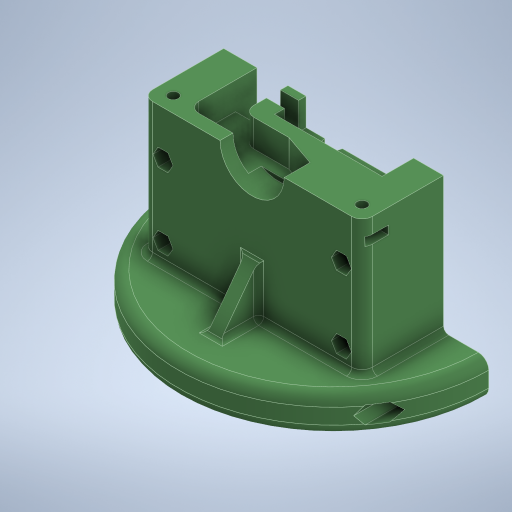
# Autodesk Inventor part: Base_1L
Saved by Autodesk Inventor 2023 (Build 270158000, 158)
## iProperties
Created: 2024-07-30
Part Number: Base_1L
Material: Generic
Document SubType Name: Modeling
Designer: Swoby
Density: 1 g/cm^3
Appearance: Default
Author: Swoby
Autodesk Inventor part; units mm, degrees
ref_plane "YZ Plane" through (0, 0, 0) normal (1, 0, 0) x (0, 1, 0)
ref_plane "XZ Plane" through (0, 0, 0) normal (0, 1, 0) x (-1, 0, 0)
ref_plane "XY Plane" through (0, 0, 0) normal (0, 0, 1) x (1, 0, 0)
sketch "Sketch1" plane through (0, 0, 0) normal (0, 0, 1) x (1, 0, 0)
  arc A0 (-42.5, 0) -> (42.5, 0) centre (0, 0) ccw
  line L0 (-42.5, 0) -> (-42.5, -52.5)
  line L1 (-42.5, -52.5) -> (42.5, -52.5)
  line L2 (42.5, -52.5) -> (42.5, 0)
  line L3 (-42.5, 0) -> (42.5, 0)
  arc A1 (42.5, 0) -> (-42.5, 0) centre (0, 0) ccw construction
  dimension "d0" = 85
  dimension "d1" = 52.5
  constraints: 8 end point, 4 point on circle, 3 perpendicular, 2 centre point, 2 tangent, 1 coincident, 1 vertical
  measures "d0" diameter of A0
  measures "d1" distance from line of L1 point (0, 0)
extrude "Extrusion1" add sketch "Sketch1" along normal blind 31.5
sketch "Sketch2" plane through (-42.5, 0, 0) normal (0, 1, 0) x (1, 0, 0)
  line L0 (31.85, -43.7) -> (73.45, -43.7)
  line L1 (73.45, -3.1) -> (31.85, -3.1)
  line L2 (35.1, -3.1) -> (49.9, -3.1)
  line L3 (49.9, -3.1) -> (49.9, -1.6)
  line L4 (49.9, -1.6) -> (35.1, -1.6)
  line L5 (35.1, -1.6) -> (35.1, -3.1)
  line L6 (37.5, -1.6) -> (47.5, -1.6)
  line L7 (47.5, -1.6) -> (47.5, 0)
  line L8 (47.5, 0) -> (37.5, 0)
  line L9 (37.5, 0) -> (37.5, -1.6)
  line L10 (85, 0) -> (0, 0) projected
  line L11 (31.85, -10.6) -> (24.75, -10.6)
  line L12 (24.75, -10.6) -> (24.75, -14.3)
  line L13 (24.75, -14.3) -> (31.85, -14.3)
  line L14 (73.45, -14.3) -> (80.55, -14.3)
  line L15 (80.55, -14.3) -> (80.55, -10.6)
  line L16 (80.55, -10.6) -> (73.45, -10.6)
  line L17 (31.85, -3.1) -> (31.85, -10.6)
  line L18 (73.45, -43.7) -> (73.45, -14.3)
  line L19 (73.45, -10.6) -> (73.45, -3.1)
  line L20 (31.85, -39.8) -> (25.85, -39.8)
  line L21 (25.85, -39.8) -> (25.85, -34.4)
  line L22 (25.85, -34.4) -> (31.85, -34.4)
  line L23 (31.85, -34.4) -> (31.85, -39.8) construction
  line L24 (31.85, -14.3) -> (31.85, -34.4)
  line L25 (31.85, -39.8) -> (31.85, -43.7)
  point P0 (42.5, 0)
  point P1 (49.9, -2.35)
  point P2 (42.5, -1.6)
  point P3 (42.5, -3.1)
  point P4 (42.5, 0)
  dimension "d4" = 14.8
  dimension "d5" = 1.5
  dimension "d6" = 10
  dimension "d7" = 1.6
  dimension "d9" = 41.6
  dimension "d10" = 40.6
  dimension "d11" = 7.5
  dimension "d12" = 3.7
  dimension "d13" = 7.1
  dimension "d14" = 7.1
  dimension "d15" = 10.65
  dimension "d16" = 3.9
  dimension "d17" = 5.4
  dimension "d18" = 6
  constraints: 50 end point, 15 parallel, 7 perpendicular, 6 horizontal, 6 midpoint, 4 point on line, 3 collinear
  measures "d4" distance from line of point (49.9, -2.35) L5
  measures "d5" distance of L2.end L3.end
  measures "d6" distance between parallel lines of L7 L9
  measures "d7" distance of L6.end L7.end
  measures "d9" distance of L1.start L1.end
  measures "d10" distance of L0.end L1.start
  measures "d11" distance of L1.end L11.start
  measures "d12" distance of L11.end L12.end
  measures "d13" distance of L11.start L11.end
  measures "d14" distance of L15.end L16.end
  measures "d15" distance from line of L17 point (42.5, -3.1)
  measures "d16" distance between parallel lines of L0 L20
  measures "d17" distance of L20.end L21.end
  measures "d18" distance of L21.end L22.end
sketch "Sketch4" plane through (-42.5, -52.5, 0) normal (0, -1, 0) x (1, 0, 0)
  line L0 (0, 31.5) -> (85, 31.5) projected
  arc A0 (-17.5, 31.5) -> (102.5, 31.5) centre (42.5, 31.5) ccw
  line L1 (102.5, 31.5) -> (-17.5, 31.5)
  arc A1 (102.5, 31.5) -> (-17.5, 31.5) centre (42.5, 31.5) ccw construction
  point P0 (42.5, 0)
  dimension "d26" = 120
  constraints: 4 point on circle, 3 midpoint, 2 centre point, 2 end point, 1 horizontal
  measures "d26" diameter of A0
extrude "Extrusion3" add sketch "Sketch4" along normal blind 14
sketch "Sketch5" plane through (0, 0, 31.5) normal (0, 0, 1) x (1, 0, 0)
  line L0 (-34.5, -17.6) -> (34.5, -17.6) construction
  line L1 (34.5, -17.6) -> (34.5, -45.5) construction
  line L2 (34.5, -45.5) -> (-34.5, -45.5) construction
  line L3 (-34.5, -45.5) -> (-34.5, -17.6) construction
  line L4 (-42.5, -52.5) -> (-60, -52.5) projected
  line L5 (-42.5, 0) -> (-42.5, -52.5) projected
  line L6 (42.5, -52.5) -> (42.5, 0) projected
  circle A0 centre (-34.5, -17.6) radius 2
  circle A1 centre (-34.5, -45.5) radius 2
  circle A2 centre (34.5, -45.5) radius 2
  circle A3 centre (34.5, -17.6) radius 2
  line L7 (-60, -52.5) -> (-60, -66.5) projected
  line L8 (60, -66.5) -> (-60, -66.5) projected
  line L9 (60, -52.5) -> (60, -66.5) projected
  line L10 (60, -52.5) -> (42.5, -52.5) projected
  line L11 (42.5, 0) -> (-42.5, 0) projected
  line L12 (42.5, 0) -> (-42.5, 0) projected
  line L13 (-60, -59.5) -> (60, -59.5) construction
  circle A4 centre (-50, -59.5) radius 2
  circle A5 centre (50, -59.5) radius 2
  point P0 (0, 0)
  dimension "d29" = 7
  dimension "d31" = 8
  dimension "d32" = 8
  dimension "d33" = 4
  dimension "d34" = 4
  dimension "d35" = 4
  dimension "d36" = 4
  dimension "d71" = 4
  dimension "d72" = 4
  dimension "d73" = 10
  dimension "d74" = 10
  dimension "d80" = 17.6
  constraints: 10 end point, 6 centre point, 4 coincident, 3 midpoint, 2 parallel, 2 point on line, 1 horizontal, 1 perpendicular
  measures "d29" distance between parallel lines of L4 L2
  measures "d31" distance between parallel lines of L5 L3
  measures "d32" distance between parallel lines of L6 L1
  measures "d33" diameter of A0
  measures "d34" diameter of A1
  measures "d35" diameter of A2
  measures "d36" diameter of A3
  measures "d71" diameter of A4
  measures "d72" diameter of A5
  measures "d73" distance from line of L7 A4.centre
  measures "d74" distance from line of L9 A5.centre
  measures "d80" distance from line of L11 L0.start
extrude "Extrusion4" cut sketch "Sketch5" against normal through all contours A0 | A1 | A2 | A3 | A4 | A5
ref_plane "Work Plane1" through (0, 0, 25.5) normal (0, 0, 1) x (1, 0, 0)
sketch "Sketch6" plane through (0, 0, 25.5) normal (0, 0, 1) x (1, 0, 0)
  circle A0 centre (-34.5, -17.6) radius 2 projected
  circle A1 centre (-34.5, -45.5) radius 2 projected
  circle A2 centre (34.5, -17.6) radius 2 projected
  circle A3 centre (34.5, -45.5) radius 2 projected
  circle A4 centre (-50, -59.5) radius 2 projected
  circle A5 centre (50, -59.5) radius 2 projected
  circle A6 centre (-34.5, -17.6) radius 2 projected
  circle A7 centre (-34.5, -17.6) radius 2 projected
  line L0 (-32.5659, -14.25) -> (-30.6318, -17.6)
  line L1 (-30.6318, -17.6) -> (-32.5659, -20.95)
  line L2 (-32.5659, -20.95) -> (-36.4341, -20.95)
  line L3 (-36.4341, -20.95) -> (-38.3682, -17.6)
  line L4 (-38.3682, -17.6) -> (-36.4341, -14.25)
  line L5 (-36.4341, -14.25) -> (-32.5659, -14.25)
  line L6 (-32.5659, -42.15) -> (-30.6318, -45.5)
  line L7 (-30.6318, -45.5) -> (-32.5659, -48.85)
  line L8 (-32.5659, -48.85) -> (-36.4341, -48.85)
  line L9 (-36.4341, -48.85) -> (-38.3682, -45.5)
  line L10 (-38.3682, -45.5) -> (-36.4341, -42.15)
  line L11 (-36.4341, -42.15) -> (-32.5659, -42.15)
  line L12 (-46.1318, -59.5) -> (-48.0659, -62.85)
  line L13 (-48.0659, -62.85) -> (-51.9341, -62.85)
  line L14 (-51.9341, -62.85) -> (-53.8682, -59.5)
  line L15 (-53.8682, -59.5) -> (-51.9341, -56.15)
  line L16 (-51.9341, -56.15) -> (-48.0659, -56.15)
  line L17 (-48.0659, -56.15) -> (-46.1318, -59.5)
  line L18 (38.3682, -45.5) -> (36.4341, -48.85)
  line L19 (36.4341, -48.85) -> (32.5659, -48.85)
  line L20 (32.5659, -48.85) -> (30.6318, -45.5)
  line L21 (30.6318, -45.5) -> (32.5659, -42.15)
  line L22 (32.5659, -42.15) -> (36.4341, -42.15)
  line L23 (36.4341, -42.15) -> (38.3682, -45.5)
  line L24 (53.8682, -59.5) -> (51.9341, -62.85)
  line L25 (51.9341, -62.85) -> (48.0659, -62.85)
  line L26 (48.0659, -62.85) -> (46.1318, -59.5)
  line L27 (46.1318, -59.5) -> (48.0659, -56.15)
  line L28 (48.0659, -56.15) -> (51.9341, -56.15)
  line L29 (51.9341, -56.15) -> (53.8682, -59.5)
  line L30 (36.4341, -14.25) -> (38.3682, -17.6)
  line L31 (38.3682, -17.6) -> (36.4341, -20.95)
  line L32 (36.4341, -20.95) -> (32.5659, -20.95)
  line L33 (32.5659, -20.95) -> (30.6318, -17.6)
  line L34 (30.6318, -17.6) -> (32.5659, -14.25)
  line L35 (32.5659, -14.25) -> (36.4341, -14.25)
  line L36 (60, -66.5) -> (-60, -66.5) projected
  line L37 (-60, -66.5) -> (60, -66.5) projected
  point P0 (0, 0)
  point P1 (-50, -62.85)
  point P2 (-50, -56.15)
  point P3 (-34.5, -48.85)
  point P4 (-34.5, -42.15)
  point P5 (50, -62.85)
  point P6 (50, -56.15)
  dimension "d85" = 6.7
  dimension "d86" = 6.7
  dimension "d87" = 6.7
  dimension "d88" = 6.7
  dimension "d89" = 6.7
  constraints: 72 end point, 6 coincident, 6 midpoint, 6 parallel, 1 point on line, 80 other
  measures "d85" distance of point (-50, -62.85) point (-50, -56.15)
  measures "d86" distance of point (-34.5, -48.85) point (-34.5, -42.15)
  measures "d87" distance between parallel lines of L2 L5
  measures "d88" distance between parallel lines of L19 L22
  measures "d89" distance of point (50, -62.85) point (50, -56.15)
extrude "Extrusion5" cut sketch "Sketch6" against normal through all contours A0 | A1 | A2 | A3 | A4 | A5 | L0 L1 L2 L3 L4 L5 | L6 L7 L8 L9 L10 L11 | L12 L13 L14 L15 L16 L17 | L18 L19 L20 L21 L22 L23 | L24 L25 L26 L27 L28 L29 | L30 L31 L32 L33 L34 L35
sketch "Sketch7" plane through (-42.5, 0, 31.5) normal (0, 1, 0) x (1, 0, 0)
  line L0 (85, 0) -> (0, 0) projected
  line L1 (85, 31.5) -> (0, 31.5) projected
  line L2 (85, 31.5) -> (0, 31.5) projected
  line L3 (85, 0) -> (0, 0) projected
  circle A0 centre (6, 25.5) radius 2
  circle A1 centre (6, 6) radius 2 construction
  circle A2 centre (79, 25.5) radius 2
  circle A3 centre (79, 6) radius 2 construction
  line L4 (85, 31.5) -> (85, 0) projected
  line L5 (0, 31.5) -> (0, 0) projected
  point P0 (42.5, 31.5)
  dimension "d46" = 4
  dimension "d47" = 4
  dimension "d48" = 4
  dimension "d49" = 4
  dimension "d50" = 6
  dimension "d52" = 6
  dimension "d54" = 6
  dimension "d56" = 6
  dimension "d81" = 6
  dimension "d82" = 6
  constraints: 4 centre point
  measures "d46" diameter of A0
  measures "d47" diameter of A1
  measures "d48" diameter of A2
  measures "d49" diameter of A3
  measures "d50" distance from line of L1 A2.centre
  measures "d52" distance from line of L0 A3.centre
  measures "d54" distance from line of L2 A0.centre
  measures "d56" distance from line of L3 A1.centre
  measures "d81" distance from line of L5 A0.centre
  measures "d82" distance from line of L4 A2.centre
extrude "Extrusion6" cut sketch "Sketch7" against normal blind 10 contours A0 | A2
ref_plane "Work Plane2" through (42.5, -6, 31.5) normal (0, 1, 0) x (1, 0, 0)
sketch "Sketch8" plane through (42.5, -6, 31.5) normal (0, 1, 0) x (1, 0, 0)
  circle A0 centre (-79, 25.5) radius 2 construction
  line L0 (-75.65, 23.5659) -> (-79, 21.6318) construction
  line L1 (-79, 21.6318) -> (-82.35, 23.5659) construction
  line L2 (-82.35, 23.5659) -> (-82.35, 27.4341) construction
  line L3 (-82.35, 27.4341) -> (-79, 29.3682) construction
  line L4 (-79, 29.3682) -> (-75.65, 27.4341) construction
  line L5 (-75.65, 27.4341) -> (-75.65, 23.5659) construction
  line L6 (-75.35, 27.6073) -> (-79, 29.7147)
  line L7 (-79, 29.7147) -> (-82.65, 27.6073)
  line L8 (-82.65, 27.6073) -> (-82.65, 23.3927)
  line L9 (-82.65, 23.3927) -> (-79, 21.2853)
  line L10 (-79, 21.2853) -> (-75.35, 23.3927)
  line L11 (-75.35, 23.3927) -> (-75.35, 27.6073)
  line L12 (17.5, 0) -> (-102.5, 0) projected
  arc A1 (17.5, 0) -> (-102.5, 0) centre (-42.5, 0) ccw projected
  line L13 (0, 31.5) -> (-85, 31.5) projected
  line L14 (-85, 31.5) -> (0, 31.5) projected
  line L15 (-85, 31.5) -> (-85, 0) projected
  line L16 (-85, 31.5) -> (-85, 0) projected
  line L17 (0, 31.5) -> (0, 0) projected
  line L18 (0, 31.5) -> (0, 0) projected
  line L19 (-6, 0) -> (-10, 0) projected
  line L20 (-75, 0) -> (-79, 0) projected
  line L21 (-6, 0) -> (-10, 0) projected
  line L22 (-75, 0) -> (-79, 0) projected
  line L23 (0, 0) -> (-85, 0) projected
  line L24 (-85, 0) -> (-102.5, 0) projected
  line L25 (17.5, 0) -> (-102.5, 0) projected
  line L26 (17.5, 0) -> (0, 0) projected
  line L27 (-6, 21.2853) -> (0, 21.2853)
  line L28 (-6, 29.7147) -> (0, 29.7147)
  line L29 (0, 21.2853) -> (0, 29.7147)
  line L30 (-79, 29.7147) -> (-85, 29.7147)
  line L31 (-85, 29.7147) -> (-85, 21.2853)
  line L32 (-79, 21.2853) -> (-85, 21.2853)
  line L33 (-9.35, 27.4341) -> (-6, 29.3682) construction
  line L34 (-6, 29.3682) -> (-2.65, 27.4341) construction
  line L35 (-2.65, 27.4341) -> (-2.65, 23.5659) construction
  line L36 (-2.65, 23.5659) -> (-6, 21.6318) construction
  line L37 (-6, 21.6318) -> (-9.35, 23.5659) construction
  line L38 (-9.35, 23.5659) -> (-9.35, 27.4341) construction
  line L39 (-9.65, 27.6073) -> (-6, 29.7147)
  line L40 (-6, 29.7147) -> (-2.35, 27.6073)
  line L41 (-2.35, 27.6073) -> (-2.35, 23.3927)
  line L42 (-2.35, 23.3927) -> (-6, 21.2853)
  line L43 (-6, 21.2853) -> (-9.65, 23.3927)
  line L44 (-9.65, 23.3927) -> (-9.65, 27.6073)
  point P0 (-42.5, 31.5)
  point P1 (-6, 25.5)
  point P2 (-11.75, 31.5)
  point P3 (-4.25, 31.5)
  point P4 (-80.75, 31.5)
  point P5 (-73.25, 31.5)
  point P6 (-11.75, 31.5)
  point P7 (-4.25, 31.5)
  point P8 (-80.75, 31.5)
  point P9 (-73.25, 31.5)
  point P10 (-6, 25.5)
  point P11 (-2.65, 25.5)
  dimension "d65" = 0.3
  dimension "d70" = 6.7
  dimension "d83" = 6.7
  dimension "d84" = 0.3
  constraints: 60 end point, 6 point on line, 3 perpendicular, 2 coincident, 2 parallel, 1 midpoint, 36 other
  measures "d65" distance between parallel lines of L4 L6
  measures "d70" distance between parallel lines of L2 L5
  measures "d83" distance from line of point (-2.65, 25.5) L38
  measures "d84" distance between parallel lines of L38 L44
extrude "Extrusion7" cut sketch "Sketch8" against normal blind 3.3 contours L11 L10 L9 L8 L7 L6 | L7 L8 L9 L32 L15 L30 | L17 L27 L42 L41 L40 L28 | L40 L41 L42 L43 L44 L39
fillet "Fillet1" radius 4 4 edges at (0, -52.5, -28.5) (42.5, -26.25, 0) (-42.5, -26.25, 0) (0, -66.5, -28.5)
mirror "Mirror1" about plane through (0, -26.25, 31.5) normal (0, 0, 1) remove original yes
extrude "Extrusion8" cut sketch "Sketch2" against normal blind 10.6 contours L25 L20 L21 L22 L24 L13 L12 L11 L17 L1 L19 L16 L15 L14 L18 L0
sketch "Sketch9" plane through (-38.5, 0, 63) normal (0, 1, 0) x (1, 0, 0)
  line L0 (27.85, 31.5) -> (69.45, 31.5) projected
  line L1 (27.85, 28.6) -> (27.85, 31.5) projected
  line L2 (21.85, 28.6) -> (27.85, 28.6) projected
  line L3 (21.85, 23.2) -> (21.85, 28.6) projected
  line L4 (27.85, 23.2) -> (21.85, 23.2) projected
  line L5 (27.85, 19.3) -> (27.85, 23.2) projected
  line L6 (69.45, 19.3) -> (27.85, 19.3) projected
  line L7 (69.45, 31.5) -> (69.45, 19.3) projected
  line L8 (21.85, 23.2) -> (8.85, 23.2)
  line L9 (8.85, 23.2) -> (8.85, 31.5)
  line L10 (8.85, 31.5) -> (20.85, 31.5)
  line L11 (20.85, 31.5) -> (20.85, 28.6)
  line L12 (20.85, 28.6) -> (21.85, 28.6)
  point P0 (38.5, 63)
  dimension "d90" = 12
  dimension "d91" = 1
  constraints: 10 end point, 4 perpendicular, 1 horizontal, 1 point on line
  measures "d90" distance of L9.end L10.end
  measures "d91" distance of L11.end L2.start
extrude "Extrusion9" cut sketch "Sketch9" against normal through all contours L3 L8 L9 L10 L11 L12
sketch "Sketch10" plane through (-38.5, 0, 63) normal (0, 1, 0) x (1, 0, 0)
  line L0 (77, 0) -> (0, 0) projected
  line L1 (38.5, 0) -> (38.5, 15.8762)
  line L2 (38.5, 0) -> (50.9, 0)
  line L3 (50.9, 0) -> (50.9, 10)
  line L4 (50.9, 10) -> (38.5, 10)
  line L5 (38.5, 10) -> (38.5, 0)
  point P0 (38.5, 63)
  point P1 (38.5, 10)
  dimension "d94" = 24.8
  dimension "d95" = 10
  constraints: 10 end point, 2 parallel, 1 horizontal, 1 midpoint, 1 perpendicular, 1 vertical
  measures "d94" diameter of L3 L1
  measures "d95" distance of L2.end L3.end
revolve "Revolution2" cut sketch "Sketch10" angle 360 about axis through (0, 0, 63) along (0, 0, -1)
sketch "Sketch11" plane through (42.5, 0, 59) normal (0, 1, 0) x (1, 0, 0)
  line L0 (-30.1, 6) -> (-30.1, -4) projected
  line L1 (-4, -4) -> (-30.1, -4) projected
  arc A0 (-4, -4) -> (0, 0) centre (-4, 0) ccw projected
  line L2 (0, 0) -> (0, 27.5) projected
  line L3 (0, 27.5) -> (-11.55, 27.5) projected
  line L4 (-11.55, 27.5) -> (-11.55, 15.3) projected
  line L5 (-11.55, 15.3) -> (-53.15, 15.3) projected
  line L6 (-53.15, 15.3) -> (-53.15, 19.2) projected
  line L7 (-53.15, 19.2) -> (-72.15, 19.2) projected
  line L8 (-72.15, 19.2) -> (-72.15, 27.5) projected
  line L9 (-72.15, 27.5) -> (-85, 27.5) projected
  line L10 (-85, 0) -> (-85, 27.5) projected
  arc A1 (-85, 0) -> (-81, -4) centre (-81, 0) ccw projected
  line L11 (-54.9, -4) -> (-81, -4) projected
  line L12 (-54.9, -4) -> (-54.9, 6) projected
  line L13 (-54.9, 6) -> (-30.1, 6) projected
  circle A2 centre (-6, 2) radius 2 projected
  circle A3 centre (-79, 2) radius 2 projected
  line L14 (-30.1, 6) -> (-42.5, 10.3)
  line L15 (-42.5, 10.3) -> (-60.15, 10.3)
  line L16 (-60.15, 27.5) -> (-60.15, 24.6) projected
  line L17 (-60.15, 24.6) -> (-53.15, 24.6) projected
  line L18 (-53.15, 24.6) -> (-53.15, 27.5) projected
  line L19 (-53.15, 27.5) -> (-60.15, 27.5) projected
  line L20 (-72.15, 19.2) -> (-72.15, 1)
  line L21 (-72.15, 1) -> (-54.9, 1)
  line L22 (-42.5, 6) -> (-42.5, 10.3)
  line L23 (-54.9, 1) -> (-42.5, 1)
  line L24 (-42.5, 1) -> (-42.5, 6)
  line L25 (-42.5, 6) -> (-54.9, 6)
  line L26 (-54.9, 6) -> (-54.9, 1)
  line L27 (-60.15, 19.2) -> (-60.15, 10.3)
  point P0 (-42.5, 59)
  dimension "d97" = 5
  dimension "d98" = 5
  dimension "d109" = 7
  constraints: 20 end point, 4 perpendicular, 2 horizontal, 2 midpoint, 2 parallel, 1 point on line, 1 vertical
  measures "d97" distance between parallel lines of L21 L13
  measures "d98" distance between parallel lines of L5 L15
  measures "d109" distance between parallel lines of L27 L6
extrude "Extrusion10" cut sketch "Sketch11" against normal up to surface (10.6 mm away) contours L13 L22 L14 | L24 L23 L12 L13 | L13 L12 L21 L20 L7 L27 L15 L22
fillet "Fillet2" radius 4 2 edges at (-29.65, -5.3, 58) (-17.65, -5.3, 48.7)
sketch "Sketch12" plane through (0, 0, 0) normal (1, 0, 0) x (0, 1, 0)
  line L0 (-52.5, 31.5) -> (-52.5, 31.5) projected
  line L1 (0, 63) -> (0, 63) projected
  line L2 (0, 63) -> (-52.5, 63) projected
  line L3 (-52.5, 63) -> (0, 63) projected
  line L4 (-45.5, 63) -> (-48.85, 63) projected
  line L5 (-42.15, 63) -> (-45.5, 63) projected
  line L6 (-45.5, 63) -> (-42.15, 63) projected
  line L7 (-48.85, 63) -> (-45.5, 63) projected
  line L8 (-17.6, 63) -> (-20.95, 63) projected
  line L9 (-14.25, 63) -> (-17.6, 63) projected
  line L10 (-17.6, 63) -> (-14.25, 63) projected
  line L11 (-20.95, 63) -> (-17.6, 63) projected
  line L12 (-42.15, 63) -> (-45.5, 63) projected
  line L13 (-45.5, 63) -> (-42.15, 63) projected
  line L14 (-48.85, 63) -> (-45.5, 63) projected
  line L15 (-45.5, 63) -> (-48.85, 63) projected
  line L16 (-17.6, 63) -> (-20.95, 63) projected
  line L17 (-14.25, 63) -> (-17.6, 63) projected
  line L18 (-17.6, 63) -> (-14.25, 63) projected
  line L19 (-20.95, 63) -> (-17.6, 63) projected
  line L20 (-52.5, 31.5) -> (-52.5, 31.5) projected
  line L21 (-52.5, 31.5) -> (-52.5, 31.5) projected
  line L22 (-52.5, 31.5) -> (-52.5, 31.5) projected
  line L23 (-52.5, 59) -> (-52.5, 31.5) projected
  line L24 (-52.5, 59) -> (-52.5, 63) projected
  line L25 (-52.5, 63) -> (-52.5, 59) projected
  line L26 (-52.5, 59) -> (-52.5, 31.5) projected
  line L27 (-52.5, 63) -> (-52.5, 78)
  line L28 (-52.5, 78) -> (-32.5, 63)
  line L29 (-52.5, 63) -> (-32.5, 63)
  point P0 (0, 0)
  dimension "d102" = 20
  dimension "d103" = 15
  constraints: 6 end point, 1 collinear, 1 point on line, 1 vertical
  measures "d102" distance of L25.start L28.end
  measures "d103" distance of L25.start L27.end
extrude "Extrusion11" add sketch "Sketch12" along normal mid plane 5
fillet "Fillet3" radius 2 12 edges at (-41.3284, -52.5, 61.8284) (-20.5, -52.5, 63) (-42.5, -52.5, 45.25) (41.3284, -52.5, 61.8284) (42.5, -52.5, 45.25) (20.5, -52.5, 63) (-2.5, -52.5, 70.5) (0, -52.5, 78) (2.5, -52.5, 70.5) (0, -32.5, 63) (-2.5, -42.5, 63) (2.5, -42.5, 63)
sketch "Sketch13" plane through (42.5, 0, 59) normal (0, 1, 0) x (1, 0, 0)
  arc A0 (-90.3638, -8.6809) -> (5.3638, -8.6809) centre (-42.5, 27.5) ccw projected
  arc A1 (3.6318, -10.8648) -> (5.3638, -8.6809) centre (-42.5, 27.5) ccw projected
  arc A2 (3.6318, -10.8648) -> (5.3638, -8.6809) centre (-42.5, 27.5) ccw projected
  arc A3 (-90.3638, -8.6809) -> (5.3638, -8.6809) centre (-42.5, 27.5) ccw projected
  arc A4 (-90.3638, -8.6809) -> (-88.6318, -10.8648) centre (-42.5, 27.5) ccw projected
  arc A5 (-90.3638, -8.6809) -> (-88.6318, -10.8648) centre (-42.5, 27.5) ccw projected
  circle A6 centre (-42.5, 27.5) radius 3.4
  point P0 (-42.5, 59)
  dimension "d110" = 6.8
  constraints: 1 centre point, 1 coincident
  measures "d110" diameter of A6
extrude "Extrusion12" cut sketch "Sketch13" against normal through all
sketch "Sketch14" plane through (0, -66.5, 31.5) normal (0, -1, 0) x (1, 0, 0)
  arc A0 (3.4, 0) -> (-3.4, 0) centre (0, 0) ccw projected
  arc A1 (3.4, 0) -> (-3.4, 0) centre (0, 0) ccw projected
  line L0 (0, 0) -> (12.9047, 12.9047) construction
  line L1 (0, 0) -> (18.25, 0) construction
  circle A2 centre (11.4905, 11.4905) radius 2
  line L2 (10.3748, 13.1504) -> (1.8031, 7.3893)
  line L3 (13.1504, 10.3748) -> (7.3893, 1.8031)
  line L4 (7.3893, 1.8031) -> (1.8031, 7.3893) construction
  line L5 (0, 0) -> (-12.9047, 12.9047) construction
  circle A3 centre (-11.4905, 11.4905) radius 2
  line L6 (-13.1504, 10.3748) -> (-7.3893, 1.8031)
  line L7 (-10.3748, 13.1504) -> (-1.8031, 7.3893)
  line L8 (-1.8031, 7.3893) -> (-7.3893, 1.8031) construction
  line L9 (0, 0) -> (-12.9047, -12.9047)
  circle A4 centre (-11.4905, -11.4905) radius 2
  line L10 (-10.3748, -13.1504) -> (-1.8031, -7.3893)
  line L11 (-13.1504, -10.3748) -> (-7.3893, -1.8031)
  line L12 (-7.3893, -1.8031) -> (-1.8031, -7.3893)
  line L13 (0, 0) -> (12.9047, -12.9047)
  circle A5 centre (11.4905, -11.4905) radius 2
  line L14 (13.1504, -10.3748) -> (7.3893, -1.8031)
  line L15 (10.3748, -13.1504) -> (1.8031, -7.3893)
  line L16 (1.8031, -7.3893) -> (7.3893, -1.8031)
  arc A6 (-1.8031, 7.3893) -> (1.8031, 7.3893) centre (0, 10.072) ccw
  arc A7 (7.3893, 1.8031) -> (6.8396, 0) centre (10.072, 0) ccw
  arc A8 (-7.3893, -1.8031) -> (-6.8396, 0) centre (-10.072, 0) ccw
  arc A9 (-6.8396, 0) -> (-7.3893, 1.8031) centre (-10.072, 0) ccw
  arc A10 (6.8396, 0) -> (7.3893, -1.8031) centre (10.072, 0) ccw
  line L17 (-6.8396, 0) -> (6.8396, 0)
  point P0 (0, -31.5)
  point P1 (0, -31.5)
  point P2 (0, -31.5)
  point P3 (4.5962, 4.5962)
  point P4 (-4.5962, 4.5962)
  point P5 (-4.5962, -4.5962)
  point P6 (4.5962, -4.5962)
  point P7 (-3.4, 0)
  dimension "d113" = 45
  dimension "d114" = 18.25
  dimension "d115" = 4
  dimension "d116" = 6.5
  dimension "d117" = 7.9
  dimension "d120" = 360
  constraints: 36 end point, 22 point on circle, 10 point on line, 9 centre point, 7 tangent, 1 coincident, 1 collinear, 1 equal length, 1 horizontal, 1 midpoint, 1 perpendicular, 53 other
  measures "d113" angle of L1 L0
  measures "d114" distance of A0.centre L0.end
  measures "d115" diameter of A2
  measures "d116" distance from line of A0.centre L4
  measures "d117" distance of L3.end L2.end
extrude "Extrusion13" cut sketch "Sketch14" against normal blind 4 contours A0 L17 A9 L6 A3 L7 A6 L2 A2 L3 A7 | A2 | A3
sketch "Sketch15" plane through (0, -66.5, 31.5) normal (0, -1, 0) x (1, 0, 0)
  line L0 (-10.3748, 13.1504) -> (-1.8031, 7.3893) projected
  arc A0 (-10.3748, 13.1504) -> (-13.1504, 10.3748) centre (-11.4905, 11.4905) ccw projected
  line L1 (-7.3893, 1.8031) -> (-13.1504, 10.3748) projected
  arc A1 (-6.8396, 0) -> (-7.3893, 1.8031) centre (-10.072, 0) ccw projected
  line L2 (-3.4, 0) -> (-6.8396, 0) projected
  arc A2 (3.4, 0) -> (-3.4, 0) centre (0, 0) ccw projected
  line L3 (6.8396, 0) -> (3.4, 0) projected
  arc A3 (7.3893, 1.8031) -> (6.8396, 0) centre (10.072, 0) ccw projected
  line L4 (13.1504, 10.3748) -> (7.3893, 1.8031) projected
  arc A4 (13.1504, 10.3748) -> (10.3748, 13.1504) centre (11.4905, 11.4905) ccw projected
  line L5 (1.8031, 7.3893) -> (10.3748, 13.1504) projected
  arc A5 (-1.8031, 7.3893) -> (1.8031, 7.3893) centre (0, 10.072) ccw projected
  line L6 (-1.5521, 7.7627) -> (-10.1238, 13.5239)
  arc A6 (-10.1238, 13.5239) -> (-13.5239, 10.1238) centre (-11.4905, 11.4905) ccw
  line L7 (-13.5239, 10.1238) -> (-7.7627, 1.5521)
  arc A7 (-7.3263, -0.45) -> (-7.7627, 1.5521) centre (-10.072, 0) ccw
  line L8 (-7.3263, -0.45) -> (-2.9155, -0.45)
  arc A8 (2.9155, -0.45) -> (-2.9155, -0.45) centre (0, 0) ccw
  line L9 (2.9155, -0.45) -> (7.3263, -0.45)
  arc A9 (7.7627, 1.5521) -> (7.3263, -0.45) centre (10.072, 0) ccw
  line L10 (7.7627, 1.5521) -> (13.5239, 10.1238)
  arc A10 (13.5239, 10.1238) -> (10.1238, 13.5239) centre (11.4905, 11.4905) ccw
  line L11 (10.1238, 13.5239) -> (1.5521, 7.7627)
  arc A11 (-1.5521, 7.7627) -> (1.5521, 7.7627) centre (0, 10.072) ccw
  point P0 (0, -31.5)
  dimension "d124" = 0.45
  constraints: 12 end point, 12 point on circle, 6 centre point, 11 other
  measures "d124" distance between parallel lines of L0 L6
extrude "Extrusion14" cut sketch "Sketch15" against normal up to surface (4 mm away)
sketch "Sketch16" plane through (0, -62.5, 31.5) normal (0, -1, 0) x (1, 0, 0)
  line L0 (7.2896, 0) -> (3.4, 0) projected
  arc A0 (7.7627, 1.5521) -> (7.2896, 0) centre (10.072, 0) ccw projected
  line L1 (13.5239, 10.1238) -> (7.7627, 1.5521) projected
  arc A1 (13.5239, 10.1238) -> (10.1238, 13.5239) centre (11.4905, 11.4905) ccw projected
  line L2 (1.5521, 7.7627) -> (10.1238, 13.5239) projected
  arc A2 (-1.5521, 7.7627) -> (1.5521, 7.7627) centre (0, 10.072) ccw projected
  line L3 (-10.1238, 13.5239) -> (-1.5521, 7.7627) projected
  arc A3 (-10.1238, 13.5239) -> (-13.5239, 10.1238) centre (-11.4905, 11.4905) ccw projected
  line L4 (-7.7627, 1.5521) -> (-13.5239, 10.1238) projected
  arc A4 (-7.2896, 0) -> (-7.7627, 1.5521) centre (-10.072, 0) ccw projected
  line L5 (-3.4, 0) -> (-7.2896, 0) projected
  arc A5 (3.4, 0) -> (-3.4, 0) centre (0, 0) ccw projected
  circle A6 centre (-11.4905, 11.4905) radius 0.5
  circle A7 centre (11.4905, 11.4905) radius 0.5
  point P0 (0, -31.5)
  dimension "d127" = 1
  dimension "d128" = 1
  constraints: 2 centre point, 2 coincident
  measures "d127" diameter of A6
  measures "d128" diameter of A7
extrude "Extrusion15" cut sketch "Sketch16" against normal blind 10 contours A6 | A7
chamfer "Chamfer1" distance 15 distance2 20 1 edges at (-29.65, -66.5, 35.65) measured on face at (-30.15, -66.5, 35.65)
chamfer "Chamfer2" distance 15 distance2 20 2 edges at (-37.15, -66.5, 39.8) (-23.15, -66.5, 39.8) measured on face at (-37.15, -66.5, 40.3) measured on face at (-23.15, -66.5, 40.3)
equation "\"d14\" = d13"
body "Solid1"
